Autodesk Inventor part; units mm, degrees
(part 2 of 2)
equation "\"allenKeyHole4_0mm\" = allenKey4_0mm + allenKeyClearance"
equation "\"allenKeyHole2_5mm\" = allenKey2_5mm + allenKeyClearance"
equation "\"allenKeyHole2_0mm\" = alleyKey2_0mm + allenKeyClearance"
equation "\"allenKeyHole3_5mm\" = allenKey3_5mm + allenKeyClearance"
equation "\"allenKeyHold1_5mm\" = allenKey1_5mm + allenKeyClearance"
equation "\"depthWiderTopUnit\" = 9.525"
equation "\"depthLowerUnit\" = 9.525"
equation "\"depthOfLetters\" = 3.175"
equation "\"outerDiameter\" = 41.148"
body "Solid1"
